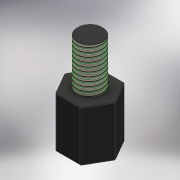
# Autodesk Inventor part: PDU Riser
Saved by Autodesk Inventor 2018 (Build 220112000, 112)
## iProperties
Created: 2018-01-07
Part Number: PDU Riser
Material: Nylon 6/6
Document SubType Name: Modeling
Designer: fbl92568
Density: 1.13 g/cm^3
Appearance: Rubber - Black
Mass: 0.18117 g
Surface Area: 2.28269 cm^2
Volume: 0.160328 cm^3
Author: fbl92568
Autodesk Inventor part; units mm, degrees
ref_plane "YZ Plane" through (0, 0, 0) normal (1, 0, 0) x (0, 1, 0)
ref_plane "XZ Plane" through (0, 0, 0) normal (0, 1, 0) x (-1, 0, 0)
ref_plane "XY Plane" through (0, 0, 0) normal (0, 0, 1) x (1, 0, 0)
sketch "Sketch1" plane through (0, 0, 0) normal (0, 0, 1) x (1, 0, 0)
  line L0 (-1.5, 2.5981) -> (1.5, 2.5981)
  line L1 (1.5, -2.5981) -> (-1.5, -2.5981)
  line L2 (1.5, 2.5981) -> (3, 0)
  line L3 (-1.5, 2.5981) -> (-3, 0)
  line L4 (-3, 0) -> (-1.5, -2.5981)
  line L5 (1.5, -2.5981) -> (3, 0)
  point P0 (0, 0)
  dimension "d1" = 3
  dimension "d2" = 3
  dimension "d3" = 120
  dimension "d4" = 3
  dimension "d5" = 120
  dimension "d6" = 120
  constraints: 12 end point, 1 equal length, 1 horizontal, 1 parallel
  measures "d1" distance of L0.start L0.end
  measures "d2" distance of L0.end L2.end
  measures "d3" angle of L0 L2
  measures "d4" distance of L1.start L1.end
  measures "d5" angle of L4 L3
  measures "d6" angle of L5 L2
extrude "Extrusion1" add sketch "Sketch1" along normal blind 6
sketch "Sketch2" plane through (0, 0, 6) normal (0, 0, 1) x (1, 0, 0)
  circle A0 centre (0, 0) radius 1.5
  dimension "d9" = 3
  constraints: 1 centre point, 1 coincident
  measures "d9" diameter of A0
extrude "Extrusion2" add sketch "Sketch2" along normal blind 5.5
sketch "Sketch3" plane through (0, 0, 0) normal (0, 0, -1) x (-1, 0, 0)
  circle A0 centre (0, 0) radius 1.4
  dimension "d12" = 2.8
  constraints: 1 centre point, 1 coincident
  measures "d12" diameter of A0
extrude "Extrusion3" cut sketch "Sketch3" against normal blind 3
thread "Thread1" size "M3x0.5" class "6H" standard "ISO Metric profile" full length
thread "Thread2" size "M3x0.5" class "6g" standard "ANSI Metric M Profile" full length
chamfer "Chamfer1" distance 0.1 angle 45 21 edges at (0, 2.5981, 0) (-1.5, 2.5981, 3) (1.5, 2.5981, 3) (3, 0, 3) (2.25, 1.299, 0) (2.25, -1.299, 0) (0, -2.5981, 0) (-2.25, -1.299, 0) (-2.25, 1.299, 0) (-3, 0, 3) (-1.5, -2.5981, 3) (1.5, -2.5981, 3) (2.25, 1.299, 6) (0, 2.5981, 6) (2.25, -1.299, 6) (-1.5, 0, 6) (0, -2.5981, 6) (-1.5, 0, 11.5) (-2.25, -1.299, 6) (-2.25, 1.299, 6) (1.4, 0, 0)
equation "\"d2\" = d1"
body "Solid1"
